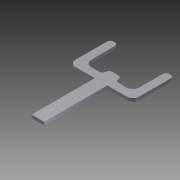
# Autodesk Inventor part: ASAP_Handle_Fixture_New2
Saved by Autodesk Inventor 2011 SP2 (Build 150309200, 309)
## iProperties
Created: 2013-02-14
Part Number: ASAP_Handle_Fixture_New2
Document SubType Name: Modeling
Designer: sungwook
Density: 1 g/cm^3
Author: sungwook
Autodesk Inventor part; units mm, degrees
ref_plane "YZ Plane" through (0, 0, 0) normal (1, 0, 0) x (0, 1, 0)
ref_plane "XZ Plane" through (0, 0, 0) normal (0, 1, 0) x (-1, 0, 0)
ref_plane "XY Plane" through (0, 0, 0) normal (0, 0, 1) x (1, 0, 0)
sketch "Sketch1" plane through (0, 0, 0) normal (0, 0, 1) x (1, 0, 0)
  line L0 (0, -25.6) -> (0, 20.6) projected
  line L1 (0, 3.5) -> (7.625, 3.5)
  line L2 (7.625, 3.5) -> (7.625, 14)
  line L3 (7.625, 14) -> (10.125, 14)
  line L4 (10.125, 14) -> (10.125, 1)
  line L5 (10.125, 1) -> (2, 1)
  line L6 (2, 1) -> (2, -19)
  line L7 (2, -19) -> (0, -19)
  line L8 (0, 3.5) -> (-7.625, 3.5)
  line L9 (-7.625, 3.5) -> (-7.625, 14)
  line L10 (-7.625, 14) -> (-10.125, 14)
  line L11 (-10.125, 14) -> (-10.125, 1)
  line L12 (-10.125, 1) -> (-2, 1)
  line L13 (-2, 1) -> (-2, -19)
  line L14 (-2, -19) -> (0, -19)
  line L15 (-2, 5.5) -> (2, 5.5)
  line L16 (2, 5.5) -> (2, 3.5)
  line L17 (2, 3.5) -> (-2, 3.5)
  line L18 (-2, 3.5) -> (-2, 5.5)
  point P0 (0, 0)
  point P1 (0, 5.5)
  dimension "d0" = 2.5
  dimension "d1" = 20.25
  dimension "d2" = 4
  dimension "d3" = 4
  dimension "d4" = 2
  dimension "d5" = 10.5
  dimension "d6" = 2.5
  dimension "d7" = 20
  constraints: 36 end point, 6 symmetric about line, 5 perpendicular, 4 parallel, 3 point on line, 1 horizontal, 1 midpoint, 1 vertical alignment
  measures "d0" distance of L3.end L2.end
  measures "d1" distance between parallel lines of L4 L11
  measures "d2" distance between parallel lines of L6 L13
  measures "d3" distance of L15.end L15.start
  measures "d4" distance of L16.end L15.end
  measures "d5" distance of L8.end L9.end
  measures "d6" distance between parallel lines of L12 L8
  measures "d7" distance from line of L6.end L5
extrude "Extrusion1" add sketch "Sketch1" along normal blind 1
fillet "Fillet1" radius 1 4 edges at (-7.625, 14, 0.5) (-10.125, 14, 0.5) (7.625, 14, 0.5) (10.125, 14, 0.5)
fillet "Fillet2" radius 1 4 edges at (-2, 5.5, 0.5) (2, 5.5, 0.5) (2, 3.5, 0.5) (-2, 3.5, 0.5)
fillet "Fillet3" radius 2 4 edges at (-10.125, 1, 0.5) (10.125, 1, 0.5) (-7.625, 3.5, 0.5) (7.625, 3.5, 0.5)
body "Solid1"
